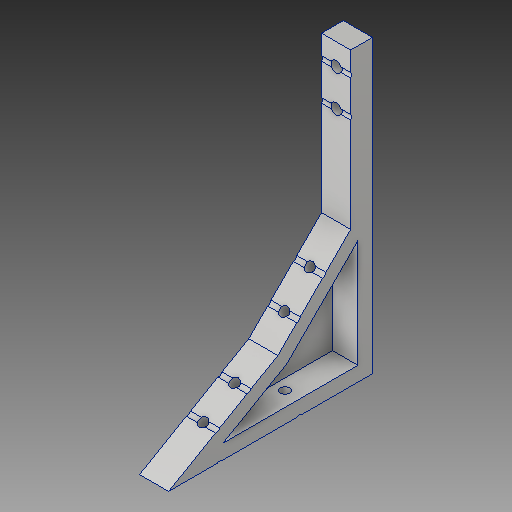
# Autodesk Inventor part: 앞판센서막이_오른쪽
Saved by Autodesk Inventor 2017 (Build 210142000, 142)
## iProperties
Part Number: 앞판센서막이_오른쪽
Material: 알루미늄 6061
Document SubType Name: Modeling
Designer: minom
Density: 2.7 g/cm^3
Appearance: 알루미늄 - 평지
Mass: 18.1843 g
Surface Area: 55.7658 cm^2
Volume: 6.73492 cm^3
Author: minom
Autodesk Inventor part; units mm, degrees
ref_plane "YZ Plane" through (0, 0, 0) normal (1, 0, 0) x (0, 1, 0)
ref_plane "XZ Plane" through (0, 0, 0) normal (0, 1, 0) x (-1, 0, 0)
sketch "스케치1" plane through (0, 0, 0) normal (1, 0, 0) x (0, 1, 0)
  line L0 (0, 0) -> (0, -30)
  line L1 (0, -30) -> (0, -50)
  line L2 (0, -50) -> (37.3205, -50)
  line L3 (0, 0) -> (17.3205, -30)
  line L4 (0, 0) -> (34.641, 0) construction
  line L5 (17.3205, -30) -> (37.3205, -50)
  line L6 (17.3205, -30) -> (43.1906, -30) construction
  line L7 (0, -30) -> (17.3205, -30)
  dimension "d0" = 30
  dimension "d1" = 20
  dimension "d2" = 60
  dimension "d3" = 45
  constraints: 16 end point, 2 horizontal, 1 collinear, 1 equal length, 1 perpendicular, 1 point on line, 1 vertical
  measures "d0" distance of L0.start L0.end
  measures "d1" distance of L0.end L1.end
  measures "d2" angle of L3 L4
  measures "d3" angle of L5 L6
extrude "돌출1" add sketch "스케치1" along normal blind 8
sketch "스케치7" plane through (0, 0, 0) normal (-1, 0, 0) x (0, 0, 1)
  line L0 (-50, 0) -> (-56, 0)
  line L1 (-56, 0) -> (-56, 80)
  line L2 (-56, 80) -> (-50, 80)
  line L3 (-50, 80) -> (-50, 0)
  point P0 (0, 0)
  dimension "d40" = 6
  dimension "d41" = 80
  constraints: 8 end point, 2 parallel, 1 horizontal, 1 perpendicular
  measures "d40" distance of L1.end L2.end
  measures "d41" distance of L0.end L1.end
extrude "돌출7" add sketch "스케치7" against normal blind 8
sketch "스케치2" plane through (8, 0, 0) normal (1, 0, 0) x (0, 0, -1)
  line L0 (0, 0) -> (56, 0) projected
  line L1 (50, 37.3205) -> (30, 17.3205) projected
  line L2 (30, 17.3205) -> (0, 0) projected
  line L3 (32.4561, 14.1197) -> (52, 33.6637)
  line L4 (52, 33.6637) -> (52, 4)
  line L5 (52, 4) -> (14.9282, 4)
  line L6 (14.9282, 4) -> (32.4561, 14.1197)
  line L7 (56, 0) -> (56, 80) projected
  line L8 (56, 80) -> (50, 80) projected
  line L9 (50, 80) -> (50, 37.3205) projected
  dimension "d7" = 4
  dimension "d44" = 4
  dimension "d53" = 4
  constraints: 8 end point, 1 other
  measures "d7" distance between parallel lines of L1 L3
  measures "d44" distance between parallel lines of L7 L4
  measures "d53" distance between parallel lines of L2 L6
extrude "돌출2" cut sketch "스케치2" against normal blind 7 contours L3 L4 L5 L6
sketch "스케치3" plane through (0, 0, -50) normal (0, -1, 0) x (1, 0, 0)
  circle A0 centre (4, 36) radius 1.25
  circle A1 centre (4, 14) radius 1.25
  line L0 (8, 50) -> (8, 0) projected
  line L1 (0, 50) -> (0, -6) projected
  line L2 (8, 50) -> (8, -6) projected
  line L3 (0, 50) -> (8, 50) projected
  line L4 (0, -6) -> (8, -6) projected
  dimension "d10" = 2.5
  dimension "d11" = 2.5
  dimension "d12" = 4
  dimension "d13" = 4
  dimension "d14" = 14
  constraints: 2 centre point
  measures "d10" diameter of A0
  measures "d11" diameter of A1
  measures "d12" distance from line of L0 A0.centre
  measures "d13" distance from line of L1 A1.centre
  measures "d14" distance from line of L3 A0.centre
extrude "돌출3" cut sketch "스케치3" against normal blind 4.1 contours A0 | A1
sketch "스케치5" plane through (0, 17.3205, -30) normal (0, 0.7071068, 0.7071068) x (1, 0, 0)
  circle A0 centre (303.8, 8) radius 1.6 projected
  circle A1 centre (263.8, 18) radius 1.6 projected
  circle A2 centre (44, 18) radius 1.6 projected
  circle A3 centre (4, 18) radius 1.6 projected
  circle A4 centre (4, 8) radius 1.6 projected
  circle A5 centre (44, 8) radius 1.6 projected
  circle A6 centre (263.8, 8) radius 1.6 projected
  circle A7 centre (303.8, 18) radius 1.6 projected
  line L0 (-1.1, 27) -> (308.9, 27) projected
  line L1 (-1.1, 1) -> (-1.1, 27) projected
  line L2 (308.9, 1) -> (161.9, 1) projected
  line L3 (145.9, 1) -> (-1.1, 1) projected
  line L4 (308.9, 27) -> (308.9, 1) projected
  circle A8 centre (4, 18) radius 1.25
  circle A9 centre (4, 8) radius 1.25
  line L5 (145.9, 1) -> (145.9, 8) projected
  arc A10 (147.9, 10) -> (145.9, 8) centre (147.9, 8) ccw projected
  line L6 (147.9, 10) -> (159.9, 10) projected
  arc A11 (161.9, 8) -> (159.9, 10) centre (159.9, 8) ccw projected
  line L7 (161.9, 8) -> (161.9, 1) projected
  circle A12 centre (111, 18) radius 1.6 projected
  circle A13 centre (196.8, 8) radius 1.6 projected
  circle A14 centre (196.8, 18) radius 1.6 projected
  circle A15 centre (111, 8) radius 1.6 projected
  point P0 (0, -33.4607)
  dimension "d22" = 2.5
  dimension "d23" = 2.5
  constraints: 2 centre point, 2 coincident
  measures "d22" diameter of A8
  measures "d23" diameter of A9
extrude "돌출5" cut sketch "스케치5" against normal blind 4.1 contours A8 | A9
sketch "스케치8" plane through (0, 37.3205, -50) normal (0, 0, 1) x (1, 0, 0)
  circle A0 centre (4, 36.6795) radius 1.5 projected
  circle A1 centre (44, 36.6795) radius 1.5 projected
  circle A2 centre (263.8, 36.6795) radius 1.5 projected
  circle A3 centre (303.8, 36.6795) radius 1.5 projected
  circle A4 centre (303.8, 26.6795) radius 1.5 projected
  circle A5 centre (263.8, 26.6795) radius 1.5 projected
  circle A6 centre (44, 26.6795) radius 1.5 projected
  circle A7 centre (4, 26.6795) radius 1.5 projected
  line L0 (193.9, 5.6795) -> (113.9, 5.6795) projected
  line L1 (113.9, 5.6795) -> (113.9, 19.6795) projected
  line L2 (113.9, 19.6795) -> (193.9, 19.6795) projected
  line L3 (193.9, 19.6795) -> (193.9, 5.6795) projected
  line L4 (78.9, 19.6795) -> (78.9, 5.6795) projected
  line L5 (78.9, 5.6795) -> (8.9, 5.6795) projected
  line L6 (8.9, 5.6795) -> (8.9, 19.6795) projected
  line L7 (8.9, 19.6795) -> (78.9, 19.6795) projected
  line L8 (298.9, 5.6795) -> (228.9, 5.6795) projected
  line L9 (228.9, 5.6795) -> (228.9, 19.6795) projected
  line L10 (228.9, 19.6795) -> (298.9, 19.6795) projected
  line L11 (298.9, 19.6795) -> (298.9, 5.6795) projected
  line L12 (308.9, 42.6795) -> (308.9, 2.6795) projected
  line L13 (-1.1, 42.6795) -> (308.9, 42.6795) projected
  line L14 (-1.1, 2.6795) -> (-1.1, 42.6795) projected
  line L15 (308.9, 2.6795) -> (-1.1, 2.6795) projected
  circle A8 centre (4, 36.6795) radius 1.25
  circle A9 centre (4, 26.6795) radius 1.25
  point P0 (0, -37.3205)
  dimension "d45" = 2.5
  dimension "d46" = 2.5
  constraints: 2 centre point, 2 coincident
  measures "d45" diameter of A8
  measures "d46" diameter of A9
extrude "돌출8" cut sketch "스케치8" against normal blind 8 contours A0 | A7 | A8 | A9
ref_plane "작업 평면1" through (0, 12.6693, -21.9438) normal (0, 0.8660254, 0.5) x (1, 0, 0)
sketch "스케치9" plane through (0, 12.6693, -21.9438) normal (0, 0.8660254, 0.5) x (1, 0, 0)
  circle A0 centre (196.8, -9.8138) radius 1.5 projected
  circle A1 centre (111, 0.1862) radius 1.5 projected
  circle A2 centre (111, -9.8138) radius 1.5 projected
  circle A3 centre (196.8, 0.1862) radius 1.5 projected
  circle A4 centre (303.8, 0.1862) radius 1.5 projected
  circle A5 centre (263.8, -9.8138) radius 1.5 projected
  circle A6 centre (44, 0.1862) radius 1.5 projected
  circle A7 centre (4, 0.1862) radius 1.5 projected
  circle A8 centre (4, -9.8138) radius 1.5 projected
  circle A9 centre (44, -9.8138) radius 1.5 projected
  circle A10 centre (263.8, 0.1862) radius 1.5 projected
  circle A11 centre (303.8, -9.8138) radius 1.5 projected
  line L0 (161.9, 8.1862) -> (161.9, 1.1862) projected
  arc A12 (159.9, -0.8138) -> (161.9, 1.1862) centre (159.9, 1.1862) ccw projected
  line L1 (159.9, -0.8138) -> (147.9, -0.8138) projected
  arc A13 (145.9, 1.1862) -> (147.9, -0.8138) centre (147.9, 1.1862) ccw projected
  line L2 (145.9, 1.1862) -> (145.9, 8.1862) projected
  line L3 (-1.1, 8.1862) -> (145.9, 8.1862) projected
  line L4 (-1.1, -25.8138) -> (-1.1, 8.1862) projected
  line L5 (308.9, -25.8138) -> (-1.1, -25.8138) projected
  line L6 (308.9, 8.1862) -> (308.9, -25.8138) projected
  line L7 (161.9, 8.1862) -> (308.9, 8.1862) projected
  circle A14 centre (4, 0.1862) radius 1.25
  circle A15 centre (4, -9.8138) radius 1.25
  point P0 (0, -25.3386)
  dimension "d49" = 2.5
  dimension "d50" = 2.5
  constraints: 2 centre point, 2 coincident
  measures "d49" diameter of A14
  measures "d50" diameter of A15
extrude "돌출9" cut sketch "스케치9" against normal blind 4.1 contours A14 | A15
sketch "스케치10" plane through (0, 0, 0) normal (-1, 0, 0) x (0, 0, 1)
  line L0 (-56, 72.5) -> (-56, 75.5) projected
  line L1 (-50, 75.5) -> (-50, 72.5) projected
  line L2 (-56, 62.5) -> (-56, 65.5) projected
  line L3 (-50, 65.5) -> (-50, 62.5) projected
  line L4 (-44.6725, 26.3361) -> (-46.4402, 28.1039) projected
  line L5 (-43.6118, 30.9323) -> (-41.844, 29.1645) projected
  line L6 (-36.5407, 23.8612) -> (-34.773, 22.0935) projected
  line L7 (-37.6014, 19.2651) -> (-39.3692, 21.0328) projected
  line L8 (-36.5407, 23.8612) -> (-34.773, 22.0935) projected
  line L9 (-23.0225, 8.6733) -> (-25.1876, 9.9233) projected
  line L10 (-23.1876, 13.3874) -> (-21.0225, 12.1374) projected
  line L11 (-14.5274, 8.3874) -> (-12.3623, 7.1374) projected
  line L12 (-14.8011, 3.8111) -> (-14.7237, 4.1) projected
  line L13 (-14.8011, 3.8111) -> (-15.1282, 4) projected
  line L14 (-14.9282, 4) -> (-15.1282, 4) projected
  line L15 (-14.9282, 4) -> (-14.9282, 4) projected
  line L16 (-15.1282, 4) -> (-14.9282, 4) projected
  line L17 (-15.1282, 4) -> (-14.8011, 3.8111) projected
  line L18 (-14.7237, 4.1) -> (-14.8011, 3.8111) projected
  line L19 (-14.7237, 4.1) -> (-14.7237, 4.1) projected
  line L20 (-14.8011, 3.8111) -> (-14.7237, 4.1) projected
  line L21 (-14.7237, 4.1) -> (-14.7237, 4.1) projected
  line L22 (-14.7237, 4.1) -> (-14.8011, 3.8111) projected
  line L23 (-14.8011, 3.8111) -> (-15.1282, 4) projected
  line L24 (-15.1282, 4) -> (-15.1282, 4) projected
  line L25 (-15.1282, 4) -> (-14.8011, 3.8111) projected
  line L26 (-12.75, 0) -> (-15.25, 0) projected
  line L27 (-37.25, 4) -> (-34.75, 4) projected
  line L28 (-34.75, 0) -> (-37.25, 0) projected
  arc A0 (-50, 74.6614) -> (-50, 73.3386) centre (-49.25, 74) ccw
  arc A1 (-50, 64.6614) -> (-50, 63.3386) centre (-49.25, 64) ccw
  arc A2 (-43.1956, 30.5161) -> (-42.2602, 29.5807) centre (-42.1976, 30.5788) ccw
  arc A3 (-36.1246, 23.4451) -> (-35.1891, 22.5097) centre (-35.1265, 23.5077) ccw
  arc A4 (-22.6779, 13.0931) -> (-21.5323, 12.4317) centre (-21.7301, 13.4119) ccw
  arc A5 (-14.0176, 8.0931) -> (-12.872, 7.4317) centre (-13.0698, 8.4119) ccw
  arc A6 (-13.3386, 0) -> (-14.6614, 0) centre (-14, -0.75) ccw
  arc A7 (-35.3386, 0) -> (-36.6614, 0) centre (-36, -0.75) ccw
  point P0 (0, 0)
  dimension "d54" = 2
  dimension "d55" = 2
  dimension "d56" = 2
  dimension "d57" = 2
  dimension "d58" = 2
  dimension "d59" = 2
  dimension "d60" = 2
  dimension "d61" = 2
  dimension "d62" = 0.75
  dimension "d63" = 0.75
  dimension "d64" = 0.75
  dimension "d65" = 0.75
  dimension "d66" = 0.75
  dimension "d67" = 0.75
  dimension "d68" = 0.75
  dimension "d69" = 0.75
  constraints: 16 point on circle, 16 point on line, 8 centre point
  measures "d54" diameter of A0
  measures "d55" diameter of A1
  measures "d56" diameter of A2
  measures "d57" diameter of A3
  measures "d58" diameter of A4
  measures "d59" diameter of A5
  measures "d60" diameter of A6
  measures "d61" diameter of A7
  measures "d62" distance from line of L28 A7.centre
  measures "d63" distance from line of L26 A6.centre
  measures "d64" distance from line of L11 A5.centre
  measures "d65" distance from line of L10 A4.centre
  measures "d66" distance from line of L6 A3.centre
  measures "d67" distance from line of L5 A2.centre
  measures "d68" distance from line of L3 A1.centre
  measures "d69" distance from line of L1 A0.centre
extrude "돌출10" cut sketch "스케치10" against normal blind 8
